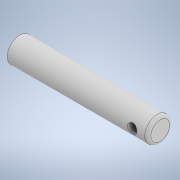
# Autodesk Inventor part: piston
Saved by Autodesk Inventor 2020 (Build 240168000, 168)
## iProperties
Created: 2022-05-04
Part Number: piston
Material: Genérico
Document SubType Name: Modeling
Designer: 19710060
Density: 1 g/cm^3
Appearance: Padrão
Author: 19710060
Autodesk Inventor part; units mm, degrees
ref_plane "YZ Plane" through (0, 0, 0) normal (1, 0, 0) x (0, 1, 0)
ref_plane "XZ Plane" through (0, 0, 0) normal (0, 1, 0) x (-1, 0, 0)
sketch "Esboço1" plane through (0, 0, 0) normal (1, 0, 0) x (0, 1, 0)
  circle A0 centre (0, 0) radius 4
  dimension "d0" = 8
  constraints: 1 centre point, 1 coincident
  measures "d0" diameter of A0
extrude "Extrusão1" add sketch "Esboço1" along normal blind 45
fillet "Arredondamento1" radius 1 1 edges at (45, -4, 0)
ref_plane "Plano de trabalho1" through (0, 0, 4) normal (0, 0, 1) x (1, 0, 0)
sketch "Esboço2" plane through (0, 0, 4) normal (0, 0, 1) x (1, 0, 0)
  line L0 (45, 3) -> (45, -3) projected
  line L1 (45, 0) -> (40, 0)
  point P0 (0, 0)
  dimension "d5" = 5
  constraints: 2 end point, 1 horizontal, 1 midpoint
  measures "d5" distance of L1.start L1.end
hole "Furo1" at (40, 0, 4) direction (0, 0, -1) diameter 3 end through all
